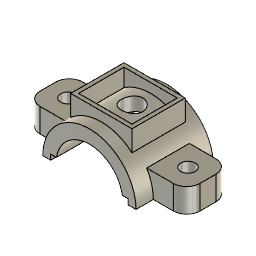
Day#15 3D Model1 v1 (Autodesk Fusion 360 design; units mm, degrees)
Autodesk Fusion 360 part; units mm, degrees
sketch "Sketch1" plane through (0, 0, 0) normal (0, 1, 0) x (1, 0, 0)
  circle A0 centre (0, 0) radius 35
  line L0 (-35, 0) -> (35, 0)
  circle A1 centre (0, 0) radius 25
  line L1 (-29, -4) -> (29, -4)
  line L2 (29, -4) -> (29, 0)
  line L3 (29, 0) -> (-29, 0)
  line L4 (-29, 0) -> (-29, -4)
  line L5 (0, -1.75) -> (0, -22.5)
  line L6 (29, 4) -> (-29, 4)
  line L7 (-29, 4) -> (-29, -4)
  line L8 (-29, -4) -> (29, -4)
  line L9 (29, -4) -> (29, 4)
  line L10 (29, 4) -> (-29, -4) construction
  line L11 (-29, 4) -> (29, -4) construction
  dimension "d1" = 70
  dimension "d4" = 50
  dimension "d5" = 58
  dimension "d6" = 4
  dimension "d7" = 58
  dimension "d8" = 8
  constraint coincident A0.centre A1.centre
  constraint coincident A0 L0.start
  constraint coincident A0 L0.end
  constraint horizontal L0
  constraint coincident A0.centre L0
  constraint horizontal L1
  constraint vertical L2
  constraint horizontal L3
  constraint vertical L4
  constraint coincident A0.centre L3
  constraint symmetric L2 L4 L5
  constraint horizontal L6
  constraint perpendicular L6 L7
  constraint parallel L6 L8
  constraint parallel L7 L9
  constraint coincident L10 A0.centre
  constraint coincident L11 A0.centre
  measures "d1" diameter of A0
  measures "d4" diameter of A1
  measures "d5" distance of L1.start L1.end
  measures "d6" distance of L1.start L3.end
  measures "d7" distance of L1.start L1.end
  measures "d8" distance of L6.end L1.start
extrude "Extrude1" add sketch "Sketch1" along normal mid plane 58 contours A0 L0 A1 L1 L2 L4 L7 L8 L9
hole "Hole1" at (0, 3.0821, 35) direction (0, 0, -1) diameter 16 end through all
ref_plane "WorkPlane1" through (60, 0, 0) normal (1, 0, 0) x (0, 1, 0)
sketch "Sketch2" plane through (60, 0, 0) normal (1, 0, 0) x (0, 1, 0)
  line L0 (16, 18) -> (-16, 18)
  line L1 (-16, 18) -> (-16, 0)
  line L2 (-16, 0) -> (16, 0)
  line L3 (16, 0) -> (16, 18)
  line L4 (16, 18) -> (-16, 0) construction
  line L5 (-16, 18) -> (16, 0) construction
  point P0 (0, 9)
  dimension "d12" = 32
  dimension "d13" = 18
  constraint horizontal L0
  constraint perpendicular L0 L1
  constraint parallel L0 L2
  constraint parallel L1 L3
  constraint coincident L4 P0
  constraint coincident L5 P0
  constraint vertical origin P0
  constraint coincident origin L2
  measures "d12" distance of L1.end L2.end
  measures "d13" distance of L0.end L1.end
extrude "Extrude2" add sketch "Sketch2" along normal up to surface end surface at (34.9565, 9.6667, 1.7446)
fillet "Fillet1" radius 10 2 edges at (60, -16, 9) (60, 16, 9)
hole "Hole2" at (45, 0, 18) direction (0, 0, -1) diameter 11 end through all
mirror "Mirror1" about plane through (0, 0, 0) normal (1, 0, 0) of "Extrude2", "Fillet1", "Hole2"
ref_plane "WorkPlane2" through (0, 0, 42) normal (0, 0, 1) x (1, 0, 0)
sketch "Sketch3" plane through (0, 0, 42) normal (0, 0, 1) x (1, 0, 0)
  line L0 (-23, 20) -> (23, 20)
  line L1 (23, 20) -> (23, -20)
  line L2 (23, -20) -> (-23, -20)
  line L3 (-23, -20) -> (-23, 20)
  line L4 (-23, 20) -> (23, -20) construction
  line L5 (23, 20) -> (-23, -20) construction
  dimension "d25" = 46
  dimension "d26" = 40
  constraint horizontal L0
  constraint perpendicular L0 L1
  constraint parallel L0 L2
  constraint parallel L1 L3
  constraint coincident L4 origin
  constraint coincident L5 origin
  measures "d25" distance of L1.end L2.end
  measures "d26" distance of L0.end L1.end
extrude "Extrude3" add sketch "Sketch3" along normal up to surface thin wall 3 inside end surface at (27.2431, 5.3333, 21.973)
equation "d1 = ( 35 * 2 ) * 1 mm"
equation "d4 = ( 25 * 2 ) * 1 mm"
